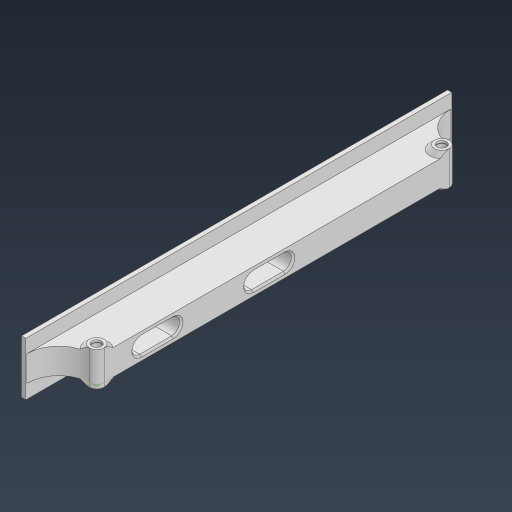
# Autodesk Inventor part: side
Saved by Autodesk Inventor 2023 (Build 270158000, 158)
## iProperties
Created: 2025-12-27
Part Number: side
Material: Generic
Document SubType Name: Modeling
Designer: szymo
Density: 1 g/cm^3
Appearance: Default
Author: szymo
Autodesk Inventor part; units mm, degrees
ref_plane "YZ Plane" through (0, 0, 0) normal (1, 0, 0) x (0, 1, 0)
ref_plane "XZ Plane" through (0, 0, 0) normal (0, 1, 0) x (-1, 0, 0)
ref_plane "XY Plane" through (0, 0, 0) normal (0, 0, 1) x (1, 0, 0)
sketch "Sketch1" plane through (0, 0, 0) normal (0, 1, 0) x (-1, 0, 0)
  circle A0 centre (0, 0) radius 3.25
  circle A1 centre (0, -162) radius 3.25
  line L0 (0, 0) -> (0, -162) construction
  line L1 (-17.8248, 3.25) -> (3.25, 3.25) construction
  line L2 (3.25, 3.25) -> (3.25, -165.25) construction
  line L3 (3.25, -165.25) -> (-25.0223, -165.25) construction
  circle A2 centre (0, 0) radius 3.5
  circle A3 centre (0, -162) radius 3.5
  dimension "d0" = 6.5
  dimension "d1" = 6.5
  dimension "d2" = 168.5
  dimension "d3" = 7
  dimension "d4" = 7
  constraints: 8 end point, 4 centre point, 3 coincident, 3 tangent, 2 perpendicular, 2 vertical
  measures "d0" diameter of A0
  measures "d1" diameter of A1
  measures "d2" distance of L1.end L2.end
  measures "d3" diameter of A2
  measures "d4" diameter of A3
extrude "Extrusion1" add sketch "Sketch1" along normal blind 16 contours A0 | A1 | A2 | A3
ref_plane "Work Plane1" through (0, 2, 0) normal (0, -1, 0) x (1, 0, 0)
sketch "Sketch2" plane through (0, 2, 0) normal (0, 1, 0) x (1, 0, 0)
  circle A0 centre (0, 0) radius 3.5 projected
  circle A1 centre (0, 162) radius 3.5 projected
  circle A2 centre (0, 0) radius 3.5 projected
  circle A3 centre (0, 0) radius 3.25
  circle A4 centre (0, 162) radius 3.5 projected
  circle A5 centre (0, 162) radius 3.25
  circle A6 centre (0, 0) radius 3.5
  circle A7 centre (0, 162) radius 3.5 projected
  circle A8 centre (0, 162) radius 3.5
  line L0 (3.5, -3.5) -> (-14.25, -3.5)
  line L1 (-14.25, -3.5) -> (-14.25, 3.5)
  line L2 (-14.25, 3.5) -> (3.5, 3.5)
  line L3 (3.5, 3.5) -> (3.5, -3.5)
  line L4 (3.5, 158.5) -> (-14.25, 158.5)
  line L5 (-14.25, 158.5) -> (-14.25, 165.5)
  line L6 (-14.25, 165.5) -> (3.5, 165.5)
  line L7 (3.5, 165.5) -> (3.5, 158.5)
  point P0 (0, 3.5)
  point P1 (0, -3.5)
  point P2 (0, 158.5)
  point P3 (0, 165.5)
  dimension "d7" = 6.5
  dimension "d8" = 6.5
  dimension "d10" = 7
  dimension "d11" = 7
  dimension "d12" = 11
  dimension "d13" = 11
  constraints: 16 end point, 6 tangent, 4 centre point, 4 coincident, 4 parallel, 2 horizontal, 2 perpendicular
  measures "d7" diameter of A3
  measures "d8" diameter of A5
  measures "d10" diameter of A6
  measures "d11" diameter of A8
  measures "d12" distance edge to line of A3 L1
  measures "d13" distance edge to line of A5 L5
extrude "Extrusion2" add sketch "Sketch2" along normal blind 12 contours A0 | A0 L0 L1 L2 | A1 | A1 L4 L5 L6 | A3 | A5
sketch "Sketch3" plane through (-14.25, 2, -165.5) normal (-1, 0, 0) x (0, 0, 1)
  line L0 (-15.5, 18.5) -> (184.5, 18.5)
  line L1 (184.5, 18.5) -> (184.5, -6.5)
  line L2 (184.5, -6.5) -> (-15.5, -6.5)
  line L3 (-15.5, -6.5) -> (-15.5, 18.5)
  line L4 (0, 0) -> (7, 0) projected
  line L5 (7, 0) -> (7, 12) projected
  line L6 (0, 12) -> (7, 12) projected
  line L7 (0, 0) -> (0, 12) projected
  line L8 (162, 0) -> (169, 0) projected
  line L9 (169, 0) -> (169, 12) projected
  line L10 (162, 12) -> (169, 12) projected
  line L11 (162, 0) -> (162, 12) projected
  point P0 (165.5, -2)
  dimension "d16" = 200
  dimension "d17" = 25
  dimension "d18" = 15.5
  dimension "d19" = 15.5
  dimension "d20" = 6.5
  dimension "d21" = 6.5
  constraints: 8 end point, 2 parallel, 1 horizontal, 1 perpendicular
  measures "d16" distance of L0.start L0.end
  measures "d17" distance of L2.end L0.start
  measures "d18" distance between parallel lines of L3 L7
  measures "d19" distance between parallel lines of L1 L9
  measures "d20" distance between parallel lines of L0 L6
  measures "d21" distance between parallel lines of L2 L4
extrude "Extrusion3" add sketch "Sketch3" along normal blind 2 contours L0 L1 L2 L3 | L7 L6 L5 L4 | L11 L10 L9 L8
sketch "Sketch4" plane through (0, 16, -162) normal (0, 1, 0) x (1, 0, 0)
  circle A0 centre (0, -162) radius 3.5 projected
  circle A1 centre (0, 0) radius 3.5 projected
  constraints: 2 coincident
hole "Hole1" at (0, 16, -162) at (0, 16, 0) direction (0, -1, 0) diameter 4 depth 5 counterbore diameter 4.5 counterbore depth 1
sketch "Sketch5" plane through (0, 0, 0) normal (0, -1, 0) x (1, 0, 0)
  circle A0 centre (0, 0) radius 3.5 projected
  circle A1 centre (0, -162) radius 3.5 projected
  circle A2 centre (0, 0) radius 2.25 projected
  circle A3 centre (0, -162) radius 2 projected
  constraints: 2 coincident
hole "Hole2" at (0, 0, 0) at (0, 0, -162) direction (0, 1, 0) diameter 4 depth 5 counterbore diameter 4.5 counterbore depth 1
sketch "Sketch7" plane through (0, 14, 0) normal (0, 1, 0) x (1, 0, 0)
  arc A0 (0, 3.5) -> (0, -3.5) centre (0, 0) ccw projected
  line L0 (0, 3.5) -> (-14.25, 3.5) projected
  line L1 (-14.25, 3.5) -> (-14.25, -3.5) projected
  line L2 (-14.25, -3.5) -> (0, -3.5) projected
  arc A1 (0, 165.5) -> (0, 158.5) centre (0, 162) ccw projected
  line L3 (0, 165.5) -> (-14.25, 165.5) projected
  line L4 (-14.25, 165.5) -> (-14.25, 158.5) projected
  line L5 (-14.25, 158.5) -> (0, 158.5) projected
  circle A2 centre (0, 162) radius 2.25 projected
  circle A3 centre (0, 162) radius 3.5 projected
  circle A4 centre (0, 0) radius 2.25 projected
  circle A5 centre (0, 0) radius 3.5 projected
  circle A6 centre (0, 0) radius 3.5 projected
  line L6 (3.5, 0) -> (3.5, 162)
  line L7 (-14.25, 3.5) -> (-14.25, -3.5) projected
  line L8 (-14.25, 3.5) -> (-14.25, 158.5)
  line L9 (-16.25, 181) -> (-16.25, -19) projected
  point P0 (0, 158.5)
  constraints: 4 end point, 2 tangent, 1 parallel, 1 point on circle, 1 vertical, 2 other
extrude "Extrusion4" add sketch "Sketch7" against normal up to surface (12 mm away) contours L0 L8 L5 A3 L6 A5
chamfer "Chamfer1" distance 2 angle 45 8 edges at (-2.4749, 2, 2.4749) (0, 2, -3.5) (-2.4749, 14, 2.4749) (0, 14, -3.5) (0, 14, -158.5) (-2.4749, 14, -164.4749) (0, 2, -158.5) (-2.4749, 2, -164.4749)
fillet "Fillet1" radius 15 2 edges at (-14.25, 8, 3.5) (-14.25, 8, -165.5)
sketch "Sketch8" plane through (3.5, 14, -4.2426) normal (1, 0, 0) x (0, 0, -1)
  line L0 (9.5074, -6) -> (32.0074, -6) construction
  line L1 (13.2574, -9.75) -> (28.2574, -9.75)
  line L2 (28.2574, -2.25) -> (13.2574, -2.25)
  arc A0 (13.2574, -2.25) -> (13.2574, -9.75) centre (13.2574, -6) ccw
  arc A1 (28.2574, -9.75) -> (28.2574, -2.25) centre (28.2574, -6) ccw
  line L3 (62.0074, -6) -> (84.5074, -6) construction
  line L4 (65.7574, -9.75) -> (80.7574, -9.75)
  line L5 (80.7574, -2.25) -> (65.7574, -2.25)
  arc A2 (65.7574, -2.25) -> (65.7574, -9.75) centre (65.7574, -6) ccw
  arc A3 (80.7574, -9.75) -> (80.7574, -2.25) centre (80.7574, -6) ccw
  line L6 (157.7574, -14) -> (157.7574, 2) projected
  line L7 (0, 0) -> (153.5147, 0) projected
  line L8 (-4.2426, -14) -> (-4.2426, 2) projected
  line L9 (153.5147, -12) -> (0, -12) projected
  line L10 (157.7574, -6) -> (-4.2426, -6)
  point P0 (-4.2426, -14)
  point P1 (20.7574, -6)
  point P2 (73.2574, -6)
  point P3 (32.0074, -6)
  dimension "d44" = 22.5
  dimension "d45" = 7.5
  dimension "d46" = 22.5
  dimension "d47" = 7.5
  dimension "d48" = 25
  dimension "d49" = 30
  constraints: 18 end point, 14 point on circle, 8 tangent, 6 point on line, 4 centre point, 4 midpoint, 2 horizontal, 2 parallel, 4 other
  measures "d44" distance of L0.start L0.end
  measures "d45" diameter of A1
  measures "d46" distance of L3.start L3.end
  measures "d47" diameter of A3
  measures "d48" distance from line of point (20.757, -6) L8
  measures "d49" distance of point (62.007, -6) point (32.007, -6)
extrude "Extrusion5" cut sketch "Sketch8" against normal through all
chamfer "Chamfer2" distance 0.8 angle 45 8 edges at (3.5, 8, -66.25) (3.5, 11.75, -77.5) (3.5, 8, -88.75) (3.5, 4.25, -77.5) (3.5, 8, -36.25) (3.5, 4.25, -25) (3.5, 8, -13.75) (3.5, 11.75, -25)
chamfer "Chamfer3" distance 2 angle 45 8 edges at (-16.25, 8, -36.25) (-16.25, 11.75, -25) (-16.25, 8, -13.75) (-16.25, 4.25, -25) (-16.25, 8, -66.25) (-16.25, 4.25, -77.5) (-16.25, 8, -88.75) (-16.25, 11.75, -77.5)
equation "\"d1\" = d0"
equation "\"d18\" = d19"
equation "\"d20\" = d21"
body "Solid1"
